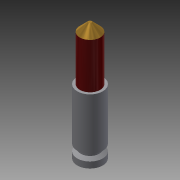
# Autodesk Inventor part: ubis
Saved by Autodesk Inventor 2014 (Build 180170000, 170)
## iProperties
Created: 2013-07-23
Part Number: ubis
Material: Generic
Document SubType Name: Modeling
Designer: employee
Density: 1 g/cm^3
Mass: 11.6315 g
Surface Area: 36.734 cm^2
Volume: 11.6315 cm^3
Appearance: Default
Author: employee
Autodesk Inventor part; units mm, degrees
ref_plane "YZ Plane" through (0, 0, 0) normal (1, 0, 0) x (0, 1, 0)
ref_plane "XZ Plane" through (0, 0, 0) normal (0, 1, 0) x (-1, 0, 0)
ref_plane "XY Plane" through (0, 0, 0) normal (0, 0, 1) x (1, 0, 0)
sketch "Sketch1" plane through (0, 0, 0) normal (0, 1, 0) x (-1, 0, 0)
  line L0 (0, 0) -> (-7.9629, 0)
  line L1 (-7.9629, 0) -> (-7.9629, 3.81)
  line L2 (-7.9629, 3.81) -> (-5.842, 5.334)
  line L3 (-5.842, 5.334) -> (-5.842, 7.239)
  line L4 (-5.842, 7.239) -> (-7.9629, 8.001)
  line L5 (-7.9629, 8.001) -> (-7.9629, 40.259)
  line L6 (-7.9629, 40.259) -> (-6.3754, 40.259)
  line L7 (-6.3754, 40.259) -> (-6.3754, 68.6656)
  line L8 (-6.3754, 68.6656) -> (-1, 74.041)
  line L9 (-1, 74.041) -> (0, 74.041)
  line L10 (0, 74.041) -> (0, 0)
  dimension "d1" = 3.81
  dimension "d3" = 74.041
  dimension "d4" = 32.258
  dimension "d5" = 0.762
  dimension "d6" = 1.524
  dimension "d7" = 4.191
  dimension "d8" = 5.842
  dimension "d9" = 7.9629
  dimension "d10" = 6.3754
  dimension "d11" = 45
  dimension "d12" = 1
  constraints: 22 end point, 5 parallel, 2 perpendicular, 1 collinear, 1 horizontal
  measures "d1" distance of L0.end L1.end
  measures "d3" distance of L9.end L0.start
  measures "d4" distance of L4.end L5.end
  measures "d5" vertical distance of L3.end L4.end
  measures "d6" vertical distance of L1.end L2.end
  measures "d7" distance of L4.end L1.end
  measures "d8" distance between parallel lines of L10 L3
  measures "d9" distance of L0.start L0.end
  measures "d10" distance between parallel lines of L10 L7
  measures "d11" angle of L10 L8
  measures "d12" distance of L8.end L9.end
revolve "Revolution1" add sketch "Sketch1" angle 360 about axis through (0, 0, 74.041) along (0, 0, -1)
body "Solid1"
